Autodesk Fusion 360 part; units mm, degrees
(part 2 of 3)
  spline S11 degree 5 poles (-7.8659, -77.7894) (-7.8562, -77.7792) (-7.8368, -77.7588) (-7.8077, -77.7282) (-7.7692, -77.6872) (-7.7213, -77.6359) (-7.6737, -77.5844) (-7.6264, -77.5328) (-7.5794, -77.481) (-7.5327, -77.4291) (-7.4862, -77.377) (-7.4401, -77.3248) (-7.3942, -77.2724) (-7.3486, -77.2199) (-7.3034, -77.1673) (-7.2584, -77.1145) (-7.2138, -77.0616) (-7.1694, -77.0085) (-7.1254, -76.9553) (-7.0816, -76.9019) (-7.0382, -76.8484) (-6.9951, -76.7947) (-6.9523, -76.7409) (-6.9099, -76.687) (-6.8678, -76.6329) (-6.826, -76.5787) (-6.7845, -76.5243) (-6.7433, -76.4698) (-6.7026, -76.4152) (-6.6621, -76.3604) (-6.622, -76.3054) (-6.5822, -76.2503) (-6.5428, -76.1951) (-6.5038, -76.1397) (-6.4651, -76.0842) (-6.4268, -76.0285) (-6.3888, -75.9727) (-6.3512, -75.9168) (-6.314, -75.8607) (-6.2772, -75.8044) (-6.2407, -75.7481) (-6.2047, -75.6915) (-6.1691, -75.6349) (-6.1338, -75.578) (-6.099, -75.5211) (-6.0646, -75.4639) (-6.0307, -75.4067) (-5.9971, -75.3493) (-5.964, -75.2917) (-5.9313, -75.234) (-5.8991, -75.1761) (-5.8673, -75.1181) (-5.8361, -75.0599) (-5.8054, -75.0016) (-5.7753, -74.9431) (-5.7456, -74.8844) (-5.7163, -74.8256) (-5.6875, -74.7667) (-5.6592, -74.7076) (-5.6315, -74.6483) (-5.6045, -74.5889) (-5.5782, -74.5292) (-5.5528, -74.4693) (-5.5282, -74.4092) (-5.5043, -74.3489) (-5.481, -74.2884) (-5.4581, -74.2278) (-5.4356, -74.1672) (-5.4137, -74.1064) (-5.3929, -74.0453) (-5.3739, -73.9839) (-5.3606, -73.9342) (-5.352, -73.8966) (-5.3468, -73.8714) (-5.3444, -73.8588) knots -1 -1 -1 -1 -1 -1 -0.98571429 -0.97142857 -0.95714286 -0.94285714 -0.92857143 -0.91428571 -0.9 -0.88571429 -0.87142857 -0.85714286 -0.84285714 -0.82857143 -0.81428571 -0.8 -0.78571429 -0.77142857 -0.75714286 -0.74285714 -0.72857143 -0.71428571 -0.7 -0.68571429 -0.67142857 -0.65714286 -0.64285714 -0.62857143 -0.61428571 -0.6 -0.58571429 -0.57142857 -0.55714286 -0.54285714 -0.52857143 -0.51428571 -0.5 -0.48571429 -0.47142857 -0.45714286 -0.44285714 -0.42857143 -0.41428571 -0.4 -0.38571429 -0.37142857 -0.35714286 -0.34285714 -0.32857143 -0.31428571 -0.3 -0.28571429 -0.27142857 -0.25714286 -0.24285714 -0.22857143 -0.21428571 -0.2 -0.18571429 -0.17142857 -0.15714286 -0.14285714 -0.12857143 -0.11428571 -0.1 -0.08571429 -0.07142857 -0.05714286 -0.04285714 -0.02857143 -0.01428571 0 0 0 0 0 0
  line L11 (-5.3444, -73.8588) -> (-5.3408, -73.8396)
  arc A23 (-3.9118, -72.8203) -> (-5.3408, -73.8396) centre (-4.0932, -74.0773) ccw
  arc A24 (-3.9118, -72.8203) -> (-3.2356, -72.9094) centre (0, -45.72) ccw
  arc A25 (-2.1191, -74.2637) -> (-3.2356, -72.9094) centre (-3.3857, -74.1705) ccw
  line L12 (-2.1191, -74.2637) -> (-2.1205, -74.2832)
  spline S12 degree 5 poles (-2.1205, -74.2832) (-2.1215, -74.2961) (-2.1231, -74.3217) (-2.1244, -74.3603) (-2.1245, -74.4117) (-2.122, -74.476) (-2.1177, -74.5403) (-2.1123, -74.6047) (-2.1063, -74.6691) (-2.0998, -74.7335) (-2.093, -74.798) (-2.0855, -74.8624) (-2.0773, -74.9269) (-2.0683, -74.9913) (-2.0583, -75.0557) (-2.0476, -75.1202) (-2.0361, -75.1846) (-2.0241, -75.249) (-2.0115, -75.3134) (-1.9985, -75.3777) (-1.985, -75.4421) (-1.971, -75.5064) (-1.9565, -75.5707) (-1.9414, -75.635) (-1.9257, -75.6992) (-1.9096, -75.7635) (-1.893, -75.8277) (-1.8759, -75.8918) (-1.8583, -75.956) (-1.8403, -76.0201) (-1.8219, -76.0842) (-1.803, -76.1482) (-1.7837, -76.2122) (-1.7639, -76.2762) (-1.7437, -76.3401) (-1.7231, -76.404) (-1.7021, -76.4678) (-1.6807, -76.5317) (-1.6589, -76.5954) (-1.6367, -76.6592) (-1.614, -76.7228) (-1.591, -76.7865) (-1.5677, -76.8501) (-1.5439, -76.9136) (-1.5197, -76.9771) (-1.4952, -77.0406) (-1.4703, -77.104) (-1.4451, -77.1673) (-1.4194, -77.2306) (-1.3935, -77.2939) (-1.3671, -77.3571) (-1.3404, -77.4202) (-1.3134, -77.4833) (-1.286, -77.5464) (-1.2582, -77.6093) (-1.2301, -77.6723) (-1.2017, -77.7351) (-1.1729, -77.7979) (-1.1438, -77.8607) (-1.1144, -77.9234) (-1.0846, -77.986) (-1.0546, -78.0486) (-1.0241, -78.1111) (-0.9934, -78.1735) (-0.9623, -78.2359) (-0.9309, -78.2982) (-0.8992, -78.3605) (-0.8672, -78.4226) (-0.8349, -78.4848) (-0.8022, -78.5468) (-0.7693, -78.6088) (-0.7426, -78.6583) (-0.7225, -78.6954) (-0.7091, -78.7202) (-0.7023, -78.7325) knots 0 0 0 0 0 0 0.01428571 0.02857143 0.04285714 0.05714286 0.07142857 0.08571429 0.1 0.11428571 0.12857143 0.14285714 0.15714286 0.17142857 0.18571429 0.2 0.21428571 0.22857143 0.24285714 0.25714286 0.27142857 0.28571429 0.3 0.31428571 0.32857143 0.34285714 0.35714286 0.37142857 0.38571429 0.4 0.41428571 0.42857143 0.44285714 0.45714286 0.47142857 0.48571429 0.5 0.51428571 0.52857143 0.54285714 0.55714286 0.57142857 0.58571429 0.6 0.61428571 0.62857143 0.64285714 0.65714286 0.67142857 0.68571429 0.7 0.71428571 0.72857143 0.74285714 0.75714286 0.77142857 0.78571429 0.8 0.81428571 0.82857143 0.84285714 0.85714286 0.87142857 0.88571429 0.9 0.91428571 0.92857143 0.94285714 0.95714286 0.97142857 0.98571429 1 1 1 1 1 1
  arc A26 (-0.7023, -78.7325) -> (0.7023, -78.7325) centre (0, -45.72) ccw
  spline S13 degree 5 poles (0.7023, -78.7325) (0.7091, -78.7202) (0.7225, -78.6954) (0.7426, -78.6583) (0.7693, -78.6088) (0.8022, -78.5468) (0.8349, -78.4848) (0.8672, -78.4226) (0.8992, -78.3605) (0.9309, -78.2982) (0.9623, -78.2359) (0.9934, -78.1735) (1.0241, -78.1111) (1.0546, -78.0486) (1.0846, -77.986) (1.1144, -77.9234) (1.1438, -77.8607) (1.1729, -77.7979) (1.2017, -77.7351) (1.2301, -77.6723) (1.2582, -77.6093) (1.286, -77.5464) (1.3134, -77.4833) (1.3404, -77.4202) (1.3671, -77.3571) (1.3935, -77.2939) (1.4194, -77.2306) (1.4451, -77.1673) (1.4703, -77.104) (1.4952, -77.0406) (1.5197, -76.9771) (1.5439, -76.9136) (1.5677, -76.8501) (1.591, -76.7865) (1.614, -76.7228) (1.6367, -76.6592) (1.6589, -76.5954) (1.6807, -76.5317) (1.7021, -76.4678) (1.7231, -76.404) (1.7437, -76.3401) (1.7639, -76.2762) (1.7837, -76.2122) (1.803, -76.1482) (1.8219, -76.0842) (1.8403, -76.0201) (1.8583, -75.956) (1.8759, -75.8918) (1.893, -75.8277) (1.9096, -75.7635) (1.9257, -75.6992) (1.9414, -75.635) (1.9565, -75.5707) (1.971, -75.5064) (1.985, -75.4421) (1.9985, -75.3777) (2.0115, -75.3134) (2.0241, -75.249) (2.0361, -75.1846) (2.0476, -75.1202) (2.0583, -75.0557) (2.0683, -74.9913) (2.0773, -74.9269) (2.0855, -74.8624) (2.093, -74.798) (2.0998, -74.7335) (2.1063, -74.6691) (2.1123, -74.6047) (2.1177, -74.5403) (2.122, -74.476) (2.1245, -74.4117) (2.1244, -74.3603) (2.1231, -74.3217) (2.1215, -74.2961) (2.1205, -74.2832) knots -1 -1 -1 -1 -1 -1 -0.98571429 -0.97142857 -0.95714286 -0.94285714 -0.92857143 -0.91428571 -0.9 -0.88571429 -0.87142857 -0.85714286 -0.84285714 -0.82857143 -0.81428571 -0.8 -0.78571429 -0.77142857 -0.75714286 -0.74285714 -0.72857143 -0.71428571 -0.7 -0.68571429 -0.67142857 -0.65714286 -0.64285714 -0.62857143 -0.61428571 -0.6 -0.58571429 -0.57142857 -0.55714286 -0.54285714 -0.52857143 -0.51428571 -0.5 -0.48571429 -0.47142857 -0.45714286 -0.44285714 -0.42857143 -0.41428571 -0.4 -0.38571429 -0.37142857 -0.35714286 -0.34285714 -0.32857143 -0.31428571 -0.3 -0.28571429 -0.27142857 -0.25714286 -0.24285714 -0.22857143 -0.21428571 -0.2 -0.18571429 -0.17142857 -0.15714286 -0.14285714 -0.12857143 -0.11428571 -0.1 -0.08571429 -0.07142857 -0.05714286 -0.04285714 -0.02857143 -0.01428571 0 0 0 0 0 0
  line L13 (2.1205, -74.2832) -> (2.1191, -74.2637)
  arc A27 (3.2356, -72.9094) -> (2.1191, -74.2637) centre (3.3857, -74.1705) ccw
  arc A28 (3.2356, -72.9094) -> (3.9118, -72.8203) centre (0, -45.72) ccw
  arc A29 (5.3408, -73.8396) -> (3.9118, -72.8203) centre (4.0932, -74.0773) ccw
  line L14 (5.3408, -73.8396) -> (5.3444, -73.8588)
  spline S14 degree 5 poles (5.3444, -73.8588) (5.3468, -73.8714) (5.352, -73.8966) (5.3606, -73.9342) (5.3739, -73.9839) (5.3929, -74.0453) (5.4137, -74.1064) (5.4356, -74.1672) (5.4581, -74.2278) (5.481, -74.2884) (5.5043, -74.3489) (5.5282, -74.4092) (5.5528, -74.4693) (5.5782, -74.5292) (5.6045, -74.5889) (5.6315, -74.6483) (5.6592, -74.7076) (5.6875, -74.7667) (5.7163, -74.8256) (5.7456, -74.8844) (5.7753, -74.9431) (5.8054, -75.0016) (5.8361, -75.0599) (5.8673, -75.1181) (5.8991, -75.1761) (5.9313, -75.234) (5.964, -75.2917) (5.9971, -75.3493) (6.0307, -75.4067) (6.0646, -75.4639) (6.099, -75.5211) (6.1338, -75.578) (6.1691, -75.6349) (6.2047, -75.6915) (6.2407, -75.7481) (6.2772, -75.8044) (6.314, -75.8607) (6.3512, -75.9168) (6.3888, -75.9727) (6.4268, -76.0285) (6.4651, -76.0842) (6.5038, -76.1397) (6.5428, -76.1951) (6.5822, -76.2503) (6.622, -76.3054) (6.6621, -76.3604) (6.7026, -76.4152) (6.7433, -76.4698) (6.7845, -76.5243) (6.826, -76.5787) (6.8678, -76.6329) (6.9099, -76.687) (6.9523, -76.7409) (6.9951, -76.7947) (7.0382, -76.8484) (7.0816, -76.9019) (7.1254, -76.9553) (7.1694, -77.0085) (7.2138, -77.0616) (7.2584, -77.1145) (7.3034, -77.1673) (7.3486, -77.2199) (7.3942, -77.2724) (7.4401, -77.3248) (7.4862, -77.377) (7.5327, -77.4291) (7.5794, -77.481) (7.6264, -77.5328) (7.6737, -77.5844) (7.7213, -77.6359) (7.7692, -77.6872) (7.8077, -77.7282) (7.8368, -77.7588) (7.8562, -77.7792) (7.8659, -77.7894) knots 0 0 0 0 0 0 0.01428571 0.02857143 0.04285714 0.05714286 0.07142857 0.08571429 0.1 0.11428571 0.12857143 0.14285714 0.15714286 0.17142857 0.18571429 0.2 0.21428571 0.22857143 0.24285714 0.25714286 0.27142857 0.28571429 0.3 0.31428571 0.32857143 0.34285714 0.35714286 0.37142857 0.38571429 0.4 0.41428571 0.42857143 0.44285714 0.45714286 0.47142857 0.48571429 0.5 0.51428571 0.52857143 0.54285714 0.55714286 0.57142857 0.58571429 0.6 0.61428571 0.62857143 0.64285714 0.65714286 0.67142857 0.68571429 0.7 0.71428571 0.72857143 0.74285714 0.75714286 0.77142857 0.78571429 0.8 0.81428571 0.82857143 0.84285714 0.85714286 0.87142857 0.88571429 0.9 0.91428571 0.92857143 0.94285714 0.95714286 0.97142857 0.98571429 1 1 1 1 1 1
  arc A30 (7.8659, -77.7894) -> (9.2227, -77.4259) centre (0, -45.72) ccw
  spline S15 degree 5 poles (9.2227, -77.4259) (9.226, -77.4122) (9.2326, -77.3848) (9.2424, -77.3438) (9.2553, -77.289) (9.2711, -77.2206) (9.2866, -77.1522) (9.3017, -77.0839) (9.3166, -77.0155) (9.3311, -76.9472) (9.3453, -76.8789) (9.3591, -76.8106) (9.3727, -76.7423) (9.3859, -76.6741) (9.3987, -76.6058) (9.4113, -76.5376) (9.4235, -76.4695) (9.4354, -76.4013) (9.4469, -76.3332) (9.4581, -76.2651) (9.4689, -76.1971) (9.4794, -76.1291) (9.4896, -76.0611) (9.4994, -75.9932) (9.5088, -75.9253) (9.5179, -75.8574) (9.5266, -75.7896) (9.535, -75.7218) (9.543, -75.6541) (9.5506, -75.5864) (9.5579, -75.5187) (9.5648, -75.4511) (9.5713, -75.3836) (9.5774, -75.3161) (9.5832, -75.2487) (9.5885, -75.1813) (9.5935, -75.114) (9.5981, -75.0468) (9.6023, -74.9796) (9.606, -74.9125) (9.6094, -74.8454) (9.6123, -74.7785) (9.6149, -74.7116) (9.6169, -74.6447) (9.6186, -74.578) (9.6198, -74.5113) (9.6206, -74.4447) (9.621, -74.3782) (9.6209, -74.3118) (9.6204, -74.2455) (9.6193, -74.1793) (9.6178, -74.1132) (9.6157, -74.0472) (9.6131, -73.9813) (9.61, -73.9156) (9.6064, -73.8499) (9.6023, -73.7844) (9.5978, -73.7189) (9.5927, -73.6536) (9.5871, -73.5884) (9.5808, -73.5234) (9.5738, -73.4586) (9.5658, -73.394) (9.5571, -73.3297) (9.5476, -73.2655) (9.5375, -73.2015) (9.5271, -73.1376) (9.5162, -73.0738) (9.5048, -73.0102) (9.4923, -72.9469) (9.478, -72.8842) (9.4647, -72.8345) (9.4534, -72.7977) (9.4452, -72.7733) (9.441, -72.7611) knots -1 -1 -1 -1 -1 -1 -0.98571429 -0.97142857 -0.95714286 -0.94285714 -0.92857143 -0.91428571 -0.9 -0.88571429 -0.87142857 -0.85714286 -0.84285714 -0.82857143 -0.81428571 -0.8 -0.78571429 -0.77142857 -0.75714286 -0.74285714 -0.72857143 -0.71428571 -0.7 -0.68571429 -0.67142857 -0.65714286 -0.64285714 -0.62857143 -0.61428571 -0.6 -0.58571429 -0.57142857 -0.55714286 -0.54285714 -0.52857143 -0.51428571 -0.5 -0.48571429 -0.47142857 -0.45714286 -0.44285714 -0.42857143 -0.41428571 -0.4 -0.38571429 -0.37142857 -0.35714286 -0.34285714 -0.32857143 -0.31428571 -0.3 -0.28571429 -0.27142857 -0.25714286 -0.24285714 -0.22857143 -0.21428571 -0.2 -0.18571429 -0.17142857 -0.15714286 -0.14285714 -0.12857143 -0.11428571 -0.1 -0.08571429 -0.07142857 -0.05714286 -0.04285714 -0.02857143 -0.01428571 0 0 0 0 0 0
  line L15 (9.441, -72.7611) -> (9.4346, -72.7427)
  arc A31 (10.1625, -71.1455) -> (9.4346, -72.7427) centre (10.6338, -72.3248) ccw
  arc A32 (10.1625, -71.1455) -> (10.7926, -70.8845) centre (0, -45.72) ccw
  arc A33 (12.4367, -71.4992) -> (10.7926, -70.8845) centre (11.2931, -72.0517) ccw
  line L16 (12.4367, -71.4992) -> (12.4452, -71.5167)
  spline S16 degree 5 poles (12.4452, -71.5167) (12.4508, -71.5283) (12.4622, -71.5514) (12.4803, -71.5854) (12.506, -71.6299) (12.5403, -71.6844) (12.5762, -71.738) (12.6131, -71.791) (12.6505, -71.8438) (12.6883, -71.8964) (12.7264, -71.9488) (12.7651, -72.0008) (12.8044, -72.0526) (12.8445, -72.1038) (12.8853, -72.1547) (12.9268, -72.2051) (12.969, -72.2551) (13.0116, -72.3049) (13.0546, -72.3544) (13.0981, -72.4036) (13.142, -72.4526) (13.1863, -72.5013) (13.231, -72.5497) (13.2762, -72.5978) (13.3219, -72.6457) (13.368, -72.6932) (13.4145, -72.7405) (13.4614, -72.7875) (13.5087, -72.8343) (13.5563, -72.8808) (13.6043, -72.9271) (13.6527, -72.9731) (13.7014, -73.0189) (13.7505, -73.0644) (13.7999, -73.1097) (13.8497, -73.1547) (13.8998, -73.1995) (13.9503, -73.244) (14.0011, -73.2883) (14.0522, -73.3324) (14.1036, -73.3763) (14.1554, -73.4199) (14.2074, -73.4633) (14.2598, -73.5064) (14.3124, -73.5493) (14.3654, -73.592) (14.4187, -73.6345) (14.4722, -73.6767) (14.5261, -73.7187) (14.5802, -73.7605) (14.6346, -73.8021) (14.6893, -73.8434) (14.7443, -73.8845) (14.7995, -73.9254) (14.855, -73.9661) (14.9108, -74.0065) (14.9669, -74.0468) (15.0232, -74.0868) (15.0797, -74.1266) (15.1366, -74.1661) (15.1937, -74.2055) (15.251, -74.2446) (15.3086, -74.2836) (15.3665, -74.3223) (15.4246, -74.3608) (15.4829, -74.399) (15.5415, -74.4371) (15.6003, -74.4749) (15.6594, -74.5125) (15.7187, -74.55) (15.7782, -74.5872) (15.826, -74.6167) (15.862, -74.6388) (15.886, -74.6535) (15.898, -74.6609) knots 0 0 0 0 0 0 0.01428571 0.02857143 0.04285714 0.05714286 0.07142857 0.08571429 0.1 0.11428571 0.12857143 0.14285714 0.15714286 0.17142857 0.18571429 0.2 0.21428571 0.22857143 0.24285714 0.25714286 0.27142857 0.28571429 0.3 0.31428571 0.32857143 0.34285714 0.35714286 0.37142857 0.38571429 0.4 0.41428571 0.42857143 0.44285714 0.45714286 0.47142857 0.48571429 0.5 0.51428571 0.52857143 0.54285714 0.55714286 0.57142857 0.58571429 0.6 0.61428571 0.62857143 0.64285714 0.65714286 0.67142857 0.68571429 0.7 0.71428571 0.72857143 0.74285714 0.75714286 0.77142857 0.78571429 0.8 0.81428571 0.82857143 0.84285714 0.85714286 0.87142857 0.88571429 0.9 0.91428571 0.92857143 0.94285714 0.95714286 0.97142857 0.98571429 1 1 1 1 1 1
  arc A34 (15.898, -74.6609) -> (17.1145, -73.9585) centre (0, -45.72) ccw
  spline S17 degree 5 poles (17.1145, -73.9585) (17.1142, -73.9444) (17.1134, -73.9163) (17.1123, -73.8741) (17.1106, -73.8179) (17.1081, -73.7477) (17.1054, -73.6777) (17.1023, -73.6077) (17.099, -73.5379) (17.0953, -73.4681) (17.0913, -73.3984) (17.0871, -73.3289) (17.0825, -73.2594) (17.0776, -73.1901) (17.0723, -73.1209) (17.0668, -73.0517) (17.0609, -72.9827) (17.0548, -72.9138) (17.0483, -72.8451) (17.0415, -72.7764) (17.0343, -72.7079) (17.0269, -72.6395) (17.0191, -72.5712) (17.011, -72.503) (17.0025, -72.435) (16.9937, -72.3671) (16.9846, -72.2993) (16.9751, -72.2317) (16.9653, -72.1642) (16.9552, -72.0968) (16.9447, -72.0296) (16.9339, -71.9625) (16.9227, -71.8956) (16.9111, -71.8288) (16.8992, -71.7622) (16.887, -71.6958) (16.8743, -71.6295) (16.8614, -71.5633) (16.848, -71.4974) (16.8343, -71.4315) (16.8202, -71.3659) (16.8057, -71.3005) (16.7908, -71.2352) (16.7755, -71.1701) (16.7599, -71.1052) (16.7438, -71.0405) (16.7273, -70.976) (16.7105, -70.9116) (16.6932, -70.8475) (16.6755, -70.7836) (16.6574, -70.7199) (16.6388, -70.6564) (16.6197, -70.5932) (16.6001, -70.5303) (16.5801, -70.4676) (16.5596, -70.4051) (16.5387, -70.3428) (16.5174, -70.2808) (16.4956, -70.219) (16.4733, -70.1575) (16.4504, -70.0963) (16.4268, -70.0356) (16.4024, -69.9752) (16.3773, -69.9153) (16.3515, -69.8558) (16.3253, -69.7966) (16.2986, -69.7375) (16.2717, -69.6787) (16.2441, -69.6203) (16.2157, -69.5624) (16.1857, -69.5055) (16.16, -69.461) (16.1395, -69.4283) (16.1253, -69.4068) (16.1181, -69.3962) knots -1 -1 -1 -1 -1 -1 -0.98571429 -0.97142857 -0.95714286 -0.94285714 -0.92857143 -0.91428571 -0.9 -0.88571429 -0.87142857 -0.85714286 -0.84285714 -0.82857143 -0.81428571 -0.8 -0.78571429 -0.77142857 -0.75714286 -0.74285714 -0.72857143 -0.71428571 -0.7 -0.68571429 -0.67142857 -0.65714286 -0.64285714 -0.62857143 -0.61428571 -0.6 -0.58571429 -0.57142857 -0.55714286 -0.54285714 -0.52857143 -0.51428571 -0.5 -0.48571429 -0.47142857 -0.45714286 -0.44285714 -0.42857143 -0.41428571 -0.4 -0.38571429 -0.37142857 -0.35714286 -0.34285714 -0.32857143 -0.31428571 -0.3 -0.28571429 -0.27142857 -0.25714286 -0.24285714 -0.22857143 -0.21428571 -0.2 -0.18571429 -0.17142857 -0.15714286 -0.14285714 -0.12857143 -0.11428571 -0.1 -0.08571429 -0.07142857 -0.05714286 -0.04285714 -0.02857143 -0.01428571 0 0 0 0 0 0
  line L17 (16.1181, -69.3962) -> (16.1071, -69.3801)
  arc A35 (16.3968, -67.6489) -> (16.1071, -69.3801) centre (17.1573, -68.666) ccw
  arc A36 (16.3968, -67.6489) -> (16.9379, -67.2337) centre (0, -45.72) ccw
  arc A37 (18.685, -67.4019) -> (16.9379, -67.2337) centre (17.7235, -68.2315) ccw
  line L18 (18.685, -67.4019) -> (18.6978, -67.4167)
  spline S18 degree 5 poles (18.6978, -67.4167) (18.7062, -67.4264) (18.7233, -67.4457) (18.7495, -67.4739) (18.7858, -67.5103) (18.8331, -67.554) (18.8816, -67.5965) (18.931, -67.6382) (18.9808, -67.6795) (19.0309, -67.7205) (19.0813, -67.7612) (19.1321, -67.8015) (19.1835, -67.8413) (19.2355, -67.8804) (19.288, -67.919) (19.3412, -67.9569) (19.3948, -67.9944) (19.4489, -68.0314) (19.5033, -68.068) (19.558, -68.1043) (19.6131, -68.1403) (19.6685, -68.1759) (19.7242, -68.2111) (19.7803, -68.2458) (19.8368, -68.2802) (19.8936, -68.3142) (19.9508, -68.3479) (20.0083, -68.3811) (20.066, -68.4141) (20.1241, -68.4467) (20.1825, -68.4789) (20.2411, -68.5109) (20.3, -68.5425) (20.3592, -68.5738) (20.4187, -68.6047) (20.4784, -68.6353) (20.5384, -68.6656) (20.5987, -68.6956) (20.6592, -68.7252) (20.72, -68.7546) (20.781, -68.7836) (20.8423, -68.8124) (20.9038, -68.8408) (20.9655, -68.8689) (21.0275, -68.8967) (21.0897, -68.9243) (21.1522, -68.9515) (21.2148, -68.9784) (21.2777, -69.0051) (21.3408, -69.0314) (21.4041, -69.0575) (21.4676, -69.0833) (21.5314, -69.1088) (21.5953, -69.134) (21.6595, -69.1589) (21.7238, -69.1835) (21.7884, -69.2079) (21.8531, -69.2319) (21.9181, -69.2557) (21.9832, -69.2792) (22.0486, -69.3025) (22.1141, -69.3254) (22.1798, -69.3481) (22.2457, -69.3705) (22.3118, -69.3927) (22.378, -69.4145) (22.4444, -69.4361) (22.5111, -69.4575) (22.5778, -69.4785) (22.6448, -69.4993) (22.7119, -69.5198) (22.7658, -69.536) (22.8062, -69.5481) (22.8333, -69.556) (22.8468, -69.56) knots 0 0 0 0 0 0 0.01428571 0.02857143 0.04285714 0.05714286 0.07142857 0.08571429 0.1 0.11428571 0.12857143 0.14285714 0.15714286 0.17142857 0.18571429 0.2 0.21428571 0.22857143 0.24285714 0.25714286 0.27142857 0.28571429 0.3 0.31428571 0.32857143 0.34285714 0.35714286 0.37142857 0.38571429 0.4 0.41428571 0.42857143 0.44285714 0.45714286 0.47142857 0.48571429 0.5 0.51428571 0.52857143 0.54285714 0.55714286 0.57142857 0.58571429 0.6 0.61428571 0.62857143 0.64285714 0.65714286 0.67142857 0.68571429 0.7 0.71428571 0.72857143 0.74285714 0.75714286 0.77142857 0.78571429 0.8 0.81428571 0.82857143 0.84285714 0.85714286 0.87142857 0.88571429 0.9 0.91428571 0.92857143 0.94285714 0.95714286 0.97142857 0.98571429 1 1 1 1 1 1
  arc A38 (22.8468, -69.56) -> (23.84, -68.5668) centre (0, -45.72) ccw
  spline S19 degree 5 poles (23.84, -68.5668) (23.836, -68.5533) (23.8281, -68.5262) (23.816, -68.4858) (23.7998, -68.4319) (23.7793, -68.3648) (23.7585, -68.2978) (23.7375, -68.2311) (23.7161, -68.1644) (23.6945, -68.098) (23.6727, -68.0318) (23.6505, -67.9657) (23.6281, -67.8998) (23.6054, -67.8341) (23.5825, -67.7686) (23.5592, -67.7032) (23.5357, -67.6381) (23.5119, -67.5731) (23.4879, -67.5084) (23.4635, -67.4438) (23.4389, -67.3795) (23.414, -67.3153) (23.3888, -67.2514) (23.3633, -67.1876) (23.3375, -67.1241) (23.3114, -67.0608) (23.2851, -66.9977) (23.2584, -66.9348) (23.2315, -66.8722) (23.2043, -66.8097) (23.1767, -66.7475) (23.1489, -66.6855) (23.1208, -66.6238) (23.0924, -66.5623) (23.0636, -66.501) (23.0346, -66.44) (23.0052, -66.3792) (22.9756, -66.3187) (22.9456, -66.2584) (22.9153, -66.1984) (22.8847, -66.1387) (22.8538, -66.0792) (22.8225, -66.02) (22.7909, -65.9611) (22.7589, -65.9025) (22.7267, -65.8441) (22.6941, -65.786) (22.6611, -65.7283) (22.6279, -65.6708) (22.5942, -65.6136) (22.5602, -65.5568) (22.5258, -65.5003) (22.4911, -65.4442) (22.4559, -65.3885) (22.4203, -65.3331) (22.3843, -65.278) (22.348, -65.2233) (22.3114, -65.1689) (22.2744, -65.1148) (22.2369, -65.0612) (22.199, -65.008) (22.1604, -64.9555) (22.1213, -64.9035) (22.0815, -64.8521) (22.0412, -64.8013) (22.0005, -64.7509) (21.9595, -64.7008) (21.9182, -64.651) (21.8765, -64.6016) (21.834, -64.5531) (21.7903, -64.5058) (21.7539, -64.4695) (21.7257, -64.4433) (21.7064, -64.4262) (21.6967, -64.4178) knots -1 -1 -1 -1 -1 -1 -0.98571429 -0.97142857 -0.95714286 -0.94285714 -0.92857143 -0.91428571 -0.9 -0.88571429 -0.87142857 -0.85714286 -0.84285714 -0.82857143 -0.81428571 -0.8 -0.78571429 -0.77142857 -0.75714286 -0.74285714 -0.72857143 -0.71428571 -0.7 -0.68571429 -0.67142857 -0.65714286 -0.64285714 -0.62857143 -0.61428571 -0.6 -0.58571429 -0.57142857 -0.55714286 -0.54285714 -0.52857143 -0.51428571 -0.5 -0.48571429 -0.47142857 -0.45714286 -0.44285714 -0.42857143 -0.41428571 -0.4 -0.38571429 -0.37142857 -0.35714286 -0.34285714 -0.32857143 -0.31428571 -0.3 -0.28571429 -0.27142857 -0.25714286 -0.24285714 -0.22857143 -0.21428571 -0.2 -0.18571429 -0.17142857 -0.15714286 -0.14285714 -0.12857143 -0.11428571 -0.1 -0.08571429 -0.07142857 -0.05714286 -0.04285714 -0.02857143 -0.01428571 0 0 0 0 0 0
  line L19 (21.6967, -64.4178) -> (21.6819, -64.405)
  arc A39 (21.5137, -62.6579) -> (21.6819, -64.405) centre (22.5115, -63.4435) ccw
  arc A40 (21.5137, -62.6579) -> (21.9289, -62.1168) centre (0, -45.72) ccw
  arc A41 (23.6601, -61.8271) -> (21.9289, -62.1168) centre (22.946, -62.8773) ccw
  line L20 (23.6601, -61.8271) -> (23.6762, -61.8381)
  spline S20 degree 5 poles (23.6762, -61.8381) (23.6868, -61.8453) (23.7083, -61.8595) (23.741, -61.88) (23.7855, -61.9057) (23.8424, -61.9357) (23.9003, -61.9641) (23.9587, -61.9917) (24.0175, -62.0186) (24.0766, -62.0453) (24.1358, -62.0715) (24.1953, -62.0973) (24.2552, -62.1224) (24.3156, -62.1468) (24.3763, -62.1704) (24.4375, -62.1933) (24.499, -62.2156) (24.5608, -62.2374) (24.6228, -62.2587) (24.6851, -62.2796) (24.7476, -62.3001) (24.8103, -62.3201) (24.8732, -62.3397) (24.9364, -62.3588) (24.9999, -62.3774) (25.0636, -62.3955) (25.1275, -62.4132) (25.1916, -62.4305) (25.256, -62.4473) (25.3205, -62.4638) (25.3852, -62.4799) (25.4501, -62.4955) (25.5152, -62.5108) (25.5805, -62.5257) (25.6459, -62.5402) (25.7115, -62.5543) (25.7774, -62.568) (25.8433, -62.5814) (25.9095, -62.5943) (25.9758, -62.607) (26.0422, -62.6192) (26.1088, -62.6311) (26.1756, -62.6427) (26.2425, -62.6539) (26.3096, -62.6647) (26.3768, -62.6752) (26.4442, -62.6853) (26.5117, -62.6951) (26.5793, -62.7046) (26.6471, -62.7137) (26.715, -62.7225) (26.783, -62.731) (26.8512, -62.7391) (26.9195, -62.7469) (26.9879, -62.7543) (27.0564, -62.7615) (27.1251, -62.7683) (27.1938, -62.7748) (27.2627, -62.7809) (27.3317, -62.7868) (27.4009, -62.7923) (27.4701, -62.7976) (27.5394, -62.8025) (27.6089, -62.8071) (27.6784, -62.8113) (27.7481, -62.8153) (27.8179, -62.819) (27.8877, -62.8223) (27.9577, -62.8254) (28.0277, -62.8281) (28.0979, -62.8306) (28.1541, -62.8323) (28.1963, -62.8334) (28.2244, -62.8342) (28.2385, -62.8345) knots 0 0 0 0 0 0 0.01428571 0.02857143 0.04285714 0.05714286 0.07142857 0.08571429 0.1 0.11428571 0.12857143 0.14285714 0.15714286 0.17142857 0.18571429 0.2 0.21428571 0.22857143 0.24285714 0.25714286 0.27142857 0.28571429 0.3 0.31428571 0.32857143 0.34285714 0.35714286 0.37142857 0.38571429 0.4 0.41428571 0.42857143 0.44285714 0.45714286 0.47142857 0.48571429 0.5 0.51428571 0.52857143 0.54285714 0.55714286 0.57142857 0.58571429 0.6 0.61428571 0.62857143 0.64285714 0.65714286 0.67142857 0.68571429 0.7 0.71428571 0.72857143 0.74285714 0.75714286 0.77142857 0.78571429 0.8 0.81428571 0.82857143 0.84285714 0.85714286 0.87142857 0.88571429 0.9 0.91428571 0.92857143 0.94285714 0.95714286 0.97142857 0.98571429 1 1 1 1 1 1
  arc A42 (28.2385, -62.8345) -> (28.9409, -61.618) centre (0, -45.72) ccw
  spline S21 degree 5 poles (28.9409, -61.618) (28.9335, -61.606) (28.9188, -61.582) (28.8967, -61.546) (28.8672, -61.4982) (28.83, -61.4387) (28.7925, -61.3794) (28.7549, -61.3203) (28.7171, -61.2615) (28.679, -61.2029) (28.6408, -61.1446) (28.6023, -61.0865) (28.5636, -61.0286) (28.5246, -60.971) (28.4855, -60.9137) (28.4461, -60.8566) (28.4066, -60.7997) (28.3668, -60.7432) (28.3268, -60.6869) (28.2865, -60.6308) (28.2461, -60.575) (28.2054, -60.5195) (28.1645, -60.4643) (28.1234, -60.4093) (28.0821, -60.3546) (28.0405, -60.3002) (27.9987, -60.2461) (27.9567, -60.1922) (27.9145, -60.1387) (27.872, -60.0854) (27.8293, -60.0324) (27.7864, -59.9798) (27.7433, -59.9274) (27.6999, -59.8754) (27.6563, -59.8236) (27.6124, -59.7722) (27.5683, -59.7211) (27.524, -59.6703) (27.4795, -59.6198) (27.4347, -59.5697) (27.3897, -59.5199) (27.3444, -59.4705) (27.2989, -59.4214) (27.2531, -59.3727) (27.2071, -59.3243) (27.1608, -59.2763) (27.1143, -59.2287) (27.0675, -59.1814) (27.0205, -59.1345) (26.9732, -59.088) (26.9257, -59.0419) (26.8778, -58.9962) (26.8297, -58.951) (26.7813, -58.9063) (26.7326, -58.862) (26.6836, -58.8181) (26.6344, -58.7746) (26.5849, -58.7316) (26.5351, -58.689) (26.4851, -58.6468) (26.4347, -58.6053) (26.3838, -58.5645) (26.3326, -58.5244) (26.2808, -58.4851) (26.2288, -58.4464) (26.1764, -58.4083) (26.1238, -58.3705) (26.071, -58.3331) (26.018, -58.2962) (25.9644, -58.2603) (25.9099, -58.226) (25.8654, -58.2003) (25.8314, -58.1822) (25.8083, -58.1708) (25.7967, -58.1652) knots -1 -1 -1 -1 -1 -1 -0.98571429 -0.97142857 -0.95714286 -0.94285714 -0.92857143 -0.91428571 -0.9 -0.88571429 -0.87142857 -0.85714286 -0.84285714 -0.82857143 -0.81428571 -0.8 -0.78571429 -0.77142857 -0.75714286 -0.74285714 -0.72857143 -0.71428571 -0.7 -0.68571429 -0.67142857 -0.65714286 -0.64285714 -0.62857143 -0.61428571 -0.6 -0.58571429 -0.57142857 -0.55714286 -0.54285714 -0.52857143 -0.51428571 -0.5 -0.48571429 -0.47142857 -0.45714286 -0.44285714 -0.42857143 -0.41428571 -0.4 -0.38571429 -0.37142857 -0.35714286 -0.34285714 -0.32857143 -0.31428571 -0.3 -0.28571429 -0.27142857 -0.25714286 -0.24285714 -0.22857143 -0.21428571 -0.2 -0.18571429 -0.17142857 -0.15714286 -0.14285714 -0.12857143 -0.11428571 -0.1 -0.08571429 -0.07142857 -0.05714286 -0.04285714 -0.02857143 -0.01428571 0 0 0 0 0 0
  line L21 (25.7967, -58.1652) -> (25.7792, -58.1567)
  arc A43 (25.1645, -56.5126) -> (25.7792, -58.1567) centre (26.3317, -57.0131) ccw
  arc A44 (25.1645, -56.5126) -> (25.4255, -55.8825) centre (0, -45.72) ccw
  arc A45 (27.0227, -55.1546) -> (25.4255, -55.8825) centre (26.6048, -56.3538) ccw
  line L22 (27.0227, -55.1546) -> (27.0411, -55.161)
  spline S22 degree 5 poles (27.0411, -55.161) (27.0533, -55.1652) (27.0777, -55.1734) (27.1145, -55.1847) (27.1642, -55.198) (27.2269, -55.2123) (27.2902, -55.2248) (27.3538, -55.2362) (27.4176, -55.2471) (27.4815, -55.2575) (27.5455, -55.2676) (27.6097, -55.2771) (27.674, -55.2858) (27.7386, -55.2938) (27.8034, -55.3008) (27.8684, -55.3071) (27.9336, -55.3127) (27.9989, -55.3178) (28.0644, -55.3223) (28.1299, -55.3264) (28.1956, -55.33) (28.2613, -55.3331) (28.3272, -55.3357) (28.3932, -55.3378) (28.4593, -55.3393) (28.5255, -55.3404) (28.5918, -55.3409) (28.6582, -55.341) (28.7247, -55.3406) (28.7913, -55.3398) (28.858, -55.3386) (28.9247, -55.3369) (28.9916, -55.3349) (29.0585, -55.3323) (29.1254, -55.3294) (29.1925, -55.326) (29.2596, -55.3223) (29.3268, -55.3181) (29.394, -55.3135) (29.4613, -55.3085) (29.5287, -55.3032) (29.5961, -55.2974) (29.6636, -55.2913) (29.7311, -55.2848) (29.7987, -55.2779) (29.8664, -55.2706) (29.9341, -55.263) (30.0018, -55.255) (30.0696, -55.2466) (30.1374, -55.2379) (30.2053, -55.2288) (30.2732, -55.2194) (30.3411, -55.2096) (30.4091, -55.1994) (30.4771, -55.1889) (30.5451, -55.1781) (30.6132, -55.1669) (30.6813, -55.1554) (30.7495, -55.1435) (30.8176, -55.1313) (30.8858, -55.1187) (30.9541, -55.1059) (31.0223, -55.0927) (31.0906, -55.0791) (31.1589, -55.0653) (31.2272, -55.0511) (31.2955, -55.0366) (31.3639, -55.0217) (31.4322, -55.0066) (31.5006, -54.9911) (31.569, -54.9753) (31.6238, -54.9624) (31.6648, -54.9526) (31.6922, -54.946) (31.7059, -54.9427) knots 0 0 0 0 0 0 0.01428571 0.02857143 0.04285714 0.05714286 0.07142857 0.08571429 0.1 0.11428571 0.12857143 0.14285714 0.15714286 0.17142857 0.18571429 0.2 0.21428571 0.22857143 0.24285714 0.25714286 0.27142857 0.28571429 0.3 0.31428571 0.32857143 0.34285714 0.35714286 0.37142857 0.38571429 0.4 0.41428571 0.42857143 0.44285714 0.45714286 0.47142857 0.48571429 0.5 0.51428571 0.52857143 0.54285714 0.55714286 0.57142857 0.58571429 0.6 0.61428571 0.62857143 0.64285714 0.65714286 0.67142857 0.68571429 0.7 0.71428571 0.72857143 0.74285714 0.75714286 0.77142857 0.78571429 0.8 0.81428571 0.82857143 0.84285714 0.85714286 0.87142857 0.88571429 0.9 0.91428571 0.92857143 0.94285714 0.95714286 0.97142857 0.98571429 1 1 1 1 1 1
  arc A46 (31.7059, -54.9427) -> (32.0694, -53.5859) centre (0, -45.72) ccw
  spline S23 degree 5 poles (32.0694, -53.5859) (32.0592, -53.5762) (32.0388, -53.5568) (32.0082, -53.5277) (31.9672, -53.4892) (31.9159, -53.4413) (31.8644, -53.3937) (31.8128, -53.3464) (31.761, -53.2994) (31.7091, -53.2527) (31.657, -53.2062) (31.6048, -53.1601) (31.5524, -53.1142) (31.4999, -53.0686) (31.4473, -53.0234) (31.3945, -52.9784) (31.3416, -52.9338) (31.2885, -52.8894) (31.2353, -52.8454) (31.1819, -52.8016) (31.1284, -52.7582) (31.0747, -52.7151) (31.0209, -52.6723) (30.967, -52.6299) (30.9129, -52.5878) (30.8587, -52.546) (30.8043, -52.5045) (30.7498, -52.4633) (30.6952, -52.4226) (30.6404, -52.3821) (30.5854, -52.342) (30.5303, -52.3022) (30.4751, -52.2628) (30.4197, -52.2238) (30.3642, -52.1851) (30.3085, -52.1468) (30.2527, -52.1088) (30.1968, -52.0712) (30.1407, -52.034) (30.0844, -51.9972) (30.0281, -51.9607) (29.9715, -51.9247) (29.9149, -51.8891) (29.858, -51.8538) (29.8011, -51.819) (29.7439, -51.7846) (29.6867, -51.7507) (29.6293, -51.7171) (29.5717, -51.684) (29.514, -51.6513) (29.4561, -51.6191) (29.3981, -51.5873) (29.3399, -51.5561) (29.2816, -51.5254) (29.2231, -51.4953) (29.1644, -51.4656) (29.1056, -51.4363) (29.0467, -51.4075) (28.9876, -51.3792) (28.9283, -51.3515) (28.8689, -51.3245) (28.8092, -51.2982) (28.7493, -51.2728) (28.6892, -51.2482) (28.6289, -51.2243) (28.5684, -51.201) (28.5078, -51.1781) (28.4472, -51.1556) (28.3864, -51.1337) (28.3253, -51.1129) (28.2639, -51.0939) (28.2142, -51.0806) (28.1766, -51.072) (28.1514, -51.0668) (28.1388, -51.0644) knots -1 -1 -1 -1 -1 -1 -0.98571429 -0.97142857 -0.95714286 -0.94285714 -0.92857143 -0.91428571 -0.9 -0.88571429 -0.87142857 -0.85714286 -0.84285714 -0.82857143 -0.81428571 -0.8 -0.78571429 -0.77142857 -0.75714286 -0.74285714 -0.72857143 -0.71428571 -0.7 -0.68571429 -0.67142857 -0.65714286 -0.64285714 -0.62857143 -0.61428571 -0.6 -0.58571429 -0.57142857 -0.55714286 -0.54285714 -0.52857143 -0.51428571 -0.5 -0.48571429 -0.47142857 -0.45714286 -0.44285714 -0.42857143 -0.41428571 -0.4 -0.38571429 -0.37142857 -0.35714286 -0.34285714 -0.32857143 -0.31428571 -0.3 -0.28571429 -0.27142857 -0.25714286 -0.24285714 -0.22857143 -0.21428571 -0.2 -0.18571429 -0.17142857 -0.15714286 -0.14285714 -0.12857143 -0.11428571 -0.1 -0.08571429 -0.07142857 -0.05714286 -0.04285714 -0.02857143 -0.01428571 0 0 0 0 0 0
  line L23 (28.1388, -51.0644) -> (28.1196, -51.0608)
  arc A47 (27.1003, -49.6318) -> (28.1196, -51.0608) centre (28.3573, -49.8132) ccw
  arc A48 (27.1003, -49.6318) -> (27.1894, -48.9556) centre (0, -45.72) ccw
  arc A49 (28.5437, -47.8391) -> (27.1894, -48.9556) centre (28.4505, -49.1057) ccw
  line L24 (28.5437, -47.8391) -> (28.5632, -47.8405)
  spline S24 degree 5 poles (28.5632, -47.8405) (28.5761, -47.8415) (28.6017, -47.8431) (28.6403, -47.8444) (28.6917, -47.8445) (28.756, -47.842) (28.8203, -47.8377) (28.8847, -47.8323) (28.9491, -47.8263) (29.0135, -47.8198) (29.078, -47.813) (29.1424, -47.8055) (29.2069, -47.7973) (29.2713, -47.7883) (29.3357, -47.7783) (29.4002, -47.7676) (29.4646, -47.7561) (29.529, -47.7441) (29.5934, -47.7315) (29.6577, -47.7185) (29.7221, -47.705) (29.7864, -47.691) (29.8507, -47.6765) (29.915, -47.6614) (29.9792, -47.6457) (30.0435, -47.6296) (30.1077, -47.613) (30.1718, -47.5959) (30.236, -47.5783) (30.3001, -47.5603) (30.3642, -47.5419) (30.4282, -47.523) (30.4922, -47.5037) (30.5562, -47.4839) (30.6201, -47.4637) (30.684, -47.4431) (30.7478, -47.4221) (30.8117, -47.4007) (30.8754, -47.3789) (30.9392, -47.3567) (31.0028, -47.334) (31.0665, -47.311) (31.1301, -47.2877) (31.1936, -47.2639) (31.2571, -47.2397) (31.3206, -47.2152) (31.384, -47.1903) (31.4473, -47.1651) (31.5106, -47.1394) (31.5739, -47.1135) (31.6371, -47.0871) (31.7002, -47.0604) (31.7633, -47.0334) (31.8264, -47.006) (31.8893, -46.9782) (31.9523, -46.9501) (32.0151, -46.9217) (32.0779, -46.8929) (32.1407, -46.8638) (32.2034, -46.8344) (32.266, -46.8046) (32.3286, -46.7746) (32.3911, -46.7441) (32.4535, -46.7134) (32.5159, -46.6823) (32.5782, -46.6509) (32.6405, -46.6192) (32.7026, -46.5872) (32.7648, -46.5549) (32.8268, -46.5222) (32.8888, -46.4893) (32.9383, -46.4626) (32.9754, -46.4425) (33.0002, -46.4291) (33.0125, -46.4223) knots 0 0 0 0 0 0 0.01428571 0.02857143 0.04285714 0.05714286 0.07142857 0.08571429 0.1 0.11428571 0.12857143 0.14285714 0.15714286 0.17142857 0.18571429 0.2 0.21428571 0.22857143 0.24285714 0.25714286 0.27142857 0.28571429 0.3 0.31428571 0.32857143 0.34285714 0.35714286 0.37142857 0.38571429 0.4 0.41428571 0.42857143 0.44285714 0.45714286 0.47142857 0.48571429 0.5 0.51428571 0.52857143 0.54285714 0.55714286 0.57142857 0.58571429 0.6 0.61428571 0.62857143 0.64285714 0.65714286 0.67142857 0.68571429 0.7 0.71428571 0.72857143 0.74285714 0.75714286 0.77142857 0.78571429 0.8 0.81428571 0.82857143 0.84285714 0.85714286 0.87142857 0.88571429 0.9 0.91428571 0.92857143 0.94285714 0.95714286 0.97142857 0.98571429 1 1 1 1 1 1
  arc A50 (33.0125, -46.4223) -> (33.0125, -45.0177) centre (0, -45.72) ccw
  spline S25 degree 5 poles (33.0125, -45.0177) (33.0002, -45.0109) (32.9754, -44.9975) (32.9383, -44.9774) (32.8888, -44.9507) (32.8268, -44.9178) (32.7648, -44.8851) (32.7026, -44.8528) (32.6405, -44.8208) (32.5782, -44.7891) (32.5159, -44.7577) (32.4535, -44.7266) (32.3911, -44.6959) (32.3286, -44.6654) (32.266, -44.6354) (32.2034, -44.6056) (32.1407, -44.5762) (32.0779, -44.5471) (32.0151, -44.5183) (31.9523, -44.4899) (31.8893, -44.4618) (31.8264, -44.434) (31.7633, -44.4066) (31.7002, -44.3796) (31.6371, -44.3529) (31.5739, -44.3265) (31.5106, -44.3006) (31.4473, -44.2749) (31.384, -44.2497) (31.3206, -44.2248) (31.2571, -44.2003) (31.1936, -44.1761) (31.1301, -44.1523) (31.0665, -44.129) (31.0028, -44.106) (30.9392, -44.0833) (30.8754, -44.0611) (30.8117, -44.0393) (30.7478, -44.0179) (30.684, -43.9969) (30.6201, -43.9763) (30.5562, -43.9561) (30.4922, -43.9363) (30.4282, -43.917) (30.3642, -43.8981) (30.3001, -43.8797) (30.236, -43.8617) (30.1718, -43.8441) (30.1077, -43.827) (30.0435, -43.8104) (29.9792, -43.7943) (29.915, -43.7786) (29.8507, -43.7635) (29.7864, -43.749) (29.7221, -43.735) (29.6577, -43.7215) (29.5934, -43.7085) (29.529, -43.6959) (29.4646, -43.6839) (29.4002, -43.6724) (29.3357, -43.6617) (29.2713, -43.6517) (29.2069, -43.6427) (29.1424, -43.6345) (29.078, -43.627) (29.0135, -43.6202) (28.9491, -43.6137) (28.8847, -43.6077) (28.8203, -43.6023) (28.756, -43.598) (28.6917, -43.5955) (28.6403, -43.5956) (28.6017, -43.5969) (28.5761, -43.5985) (28.5632, -43.5995) knots -1 -1 -1 -1 -1 -1 -0.98571429 -0.97142857 -0.95714286 -0.94285714 -0.92857143 -0.91428571 -0.9 -0.88571429 -0.87142857 -0.85714286 -0.84285714 -0.82857143 -0.81428571 -0.8 -0.78571429 -0.77142857 -0.75714286 -0.74285714 -0.72857143 -0.71428571 -0.7 -0.68571429 -0.67142857 -0.65714286 -0.64285714 -0.62857143 -0.61428571 -0.6 -0.58571429 -0.57142857 -0.55714286 -0.54285714 -0.52857143 -0.51428571 -0.5 -0.48571429 -0.47142857 -0.45714286 -0.44285714 -0.42857143 -0.41428571 -0.4 -0.38571429 -0.37142857 -0.35714286 -0.34285714 -0.32857143 -0.31428571 -0.3 -0.28571429 -0.27142857 -0.25714286 -0.24285714 -0.22857143 -0.21428571 -0.2 -0.18571429 -0.17142857 -0.15714286 -0.14285714 -0.12857143 -0.11428571 -0.1 -0.08571429 -0.07142857 -0.05714286 -0.04285714 -0.02857143 -0.01428571 0 0 0 0 0 0
  line L25 (28.5632, -43.5995) -> (28.5437, -43.6009)
  arc A51 (27.1894, -42.4844) -> (28.5437, -43.6009) centre (28.4505, -42.3343) ccw
  arc A52 (27.1894, -42.4844) -> (27.1003, -41.8082) centre (0, -45.72) ccw
  arc A53 (28.1196, -40.3792) -> (27.1003, -41.8082) centre (28.3573, -41.6268) ccw
  line L26 (28.1196, -40.3792) -> (28.1388, -40.3756)
  spline S26 degree 5 poles (28.1388, -40.3756) (28.1514, -40.3732) (28.1766, -40.368) (28.2142, -40.3594) (28.2639, -40.3461) (28.3253, -40.3271) (28.3864, -40.3063) (28.4472, -40.2844) (28.5078, -40.2619) (28.5684, -40.239) (28.6289, -40.2157) (28.6892, -40.1918) (28.7493, -40.1672) (28.8092, -40.1418) (28.8689, -40.1155) (28.9283, -40.0885) (28.9876, -40.0608) (29.0467, -40.0325) (29.1056, -40.0037) (29.1644, -39.9744) (29.2231, -39.9447) (29.2816, -39.9146) (29.3399, -39.8839) (29.3981, -39.8527) (29.4561, -39.8209) (29.514, -39.7887) (29.5717, -39.756) (29.6293, -39.7229) (29.6867, -39.6893) (29.7439, -39.6554) (29.8011, -39.621) (29.858, -39.5862) (29.9149, -39.5509) (29.9715, -39.5153) (30.0281, -39.4793) (30.0844, -39.4428) (30.1407, -39.406) (30.1968, -39.3688) (30.2527, -39.3312) (30.3085, -39.2932) (30.3642, -39.2549) (30.4197, -39.2162) (30.4751, -39.1772) (30.5303, -39.1378) (30.5854, -39.098) (30.6404, -39.0579) (30.6952, -39.0174) (30.7498, -38.9767) (30.8043, -38.9355) (30.8587, -38.894) (30.9129, -38.8522) (30.967, -38.8101) (31.0209, -38.7677) (31.0747, -38.7249) (31.1284, -38.6818) (31.1819, -38.6384) (31.2353, -38.5946) (31.2885, -38.5506) (31.3416, -38.5062) (31.3945, -38.4616) (31.4473, -38.4166) (31.4999, -38.3714) (31.5524, -38.3258) (31.6048, -38.2799) (31.657, -38.2338) (31.7091, -38.1873) (31.761, -38.1406) (31.8128, -38.0936) (31.8644, -38.0463) (31.9159, -37.9987) (31.9672, -37.9508) (32.0082, -37.9123) (32.0388, -37.8832) (32.0592, -37.8638) (32.0694, -37.8541) knots 0 0 0 0 0 0 0.01428571 0.02857143 0.04285714 0.05714286 0.07142857 0.08571429 0.1 0.11428571 0.12857143 0.14285714 0.15714286 0.17142857 0.18571429 0.2 0.21428571 0.22857143 0.24285714 0.25714286 0.27142857 0.28571429 0.3 0.31428571 0.32857143 0.34285714 0.35714286 0.37142857 0.38571429 0.4 0.41428571 0.42857143 0.44285714 0.45714286 0.47142857 0.48571429 0.5 0.51428571 0.52857143 0.54285714 0.55714286 0.57142857 0.58571429 0.6 0.61428571 0.62857143 0.64285714 0.65714286 0.67142857 0.68571429 0.7 0.71428571 0.72857143 0.74285714 0.75714286 0.77142857 0.78571429 0.8 0.81428571 0.82857143 0.84285714 0.85714286 0.87142857 0.88571429 0.9 0.91428571 0.92857143 0.94285714 0.95714286 0.97142857 0.98571429 1 1 1 1 1 1
  arc A54 (32.0694, -37.8541) -> (31.7059, -36.4973) centre (0, -45.72) ccw
  spline S27 degree 5 poles (31.7059, -36.4973) (31.6922, -36.494) (31.6648, -36.4874) (31.6238, -36.4776) (31.569, -36.4647) (31.5006, -36.4489) (31.4322, -36.4334) (31.3639, -36.4183) (31.2955, -36.4034) (31.2272, -36.3889) (31.1589, -36.3747) (31.0906, -36.3609) (31.0223, -36.3473) (30.9541, -36.3341) (30.8858, -36.3213) (30.8176, -36.3087) (30.7495, -36.2965) (30.6813, -36.2846) (30.6132, -36.2731) (30.5451, -36.2619) (30.4771, -36.2511) (30.4091, -36.2406) (30.3411, -36.2304) (30.2732, -36.2206) (30.2053, -36.2112) (30.1374, -36.2021) (30.0696, -36.1934) (30.0018, -36.185) (29.9341, -36.177) (29.8664, -36.1694) (29.7987, -36.1621) (29.7311, -36.1552) (29.6636, -36.1487) (29.5961, -36.1426) (29.5287, -36.1368) (29.4613, -36.1315) (29.394, -36.1265) (29.3268, -36.1219) (29.2596, -36.1177) (29.1925, -36.114) (29.1254, -36.1106) (29.0585, -36.1077) (28.9916, -36.1051) (28.9247, -36.1031) (28.858, -36.1014) (28.7913, -36.1002) (28.7247, -36.0994) (28.6582, -36.099) (28.5918, -36.0991) (28.5255, -36.0996) (28.4593, -36.1007) (28.3932, -36.1022) (28.3272, -36.1043) (28.2613, -36.1069) (28.1956, -36.11) (28.1299, -36.1136) (28.0644, -36.1177) (27.9989, -36.1222) (27.9336, -36.1273) (27.8684, -36.1329) (27.8034, -36.1392) (27.7386, -36.1462) (27.674, -36.1542) (27.6097, -36.1629) (27.5455, -36.1724) (27.4815, -36.1825) (27.4176, -36.1929) (27.3538, -36.2038) (27.2902, -36.2152) (27.2269, -36.2277) (27.1642, -36.242) (27.1145, -36.2553) (27.0777, -36.2666) (27.0533, -36.2748) (27.0411, -36.279) knots -1 -1 -1 -1 -1 -1 -0.98571429 -0.97142857 -0.95714286 -0.94285714 -0.92857143 -0.91428571 -0.9 -0.88571429 -0.87142857 -0.85714286 -0.84285714 -0.82857143 -0.81428571 -0.8 -0.78571429 -0.77142857 -0.75714286 -0.74285714 -0.72857143 -0.71428571 -0.7 -0.68571429 -0.67142857 -0.65714286 -0.64285714 -0.62857143 -0.61428571 -0.6 -0.58571429 -0.57142857 -0.55714286 -0.54285714 -0.52857143 -0.51428571 -0.5 -0.48571429 -0.47142857 -0.45714286 -0.44285714 -0.42857143 -0.41428571 -0.4 -0.38571429 -0.37142857 -0.35714286 -0.34285714 -0.32857143 -0.31428571 -0.3 -0.28571429 -0.27142857 -0.25714286 -0.24285714 -0.22857143 -0.21428571 -0.2 -0.18571429 -0.17142857 -0.15714286 -0.14285714 -0.12857143 -0.11428571 -0.1 -0.08571429 -0.07142857 -0.05714286 -0.04285714 -0.02857143 -0.01428571 0 0 0 0 0 0
  line L27 (27.0411, -36.279) -> (27.0227, -36.2854)
  arc A55 (25.4255, -35.5575) -> (27.0227, -36.2854) centre (26.6048, -35.0862) ccw
  arc A56 (25.4255, -35.5575) -> (25.1645, -34.9274) centre (0, -45.72) ccw
  arc A57 (25.7792, -33.2833) -> (25.1645, -34.9274) centre (26.3317, -34.4269) ccw
  line L28 (25.7792, -33.2833) -> (25.7967, -33.2748)
  spline S28 degree 5 poles (25.7967, -33.2748) (25.8083, -33.2692) (25.8314, -33.2578) (25.8654, -33.2397) (25.9099, -33.214) (25.9644, -33.1797) (26.018, -33.1438) (26.071, -33.1069) (26.1238, -33.0695) (26.1764, -33.0317) (26.2288, -32.9936) (26.2808, -32.9549) (26.3326, -32.9156) (26.3838, -32.8755) (26.4347, -32.8347) (26.4851, -32.7932) (26.5351, -32.751) (26.5849, -32.7084) (26.6344, -32.6654) (26.6836, -32.6219) (26.7326, -32.578) (26.7813, -32.5337) (26.8297, -32.489) (26.8778, -32.4438) (26.9257, -32.3981) (26.9732, -32.352) (27.0205, -32.3055) (27.0675, -32.2586) (27.1143, -32.2113) (27.1608, -32.1637) (27.2071, -32.1157) (27.2531, -32.0673) (27.2989, -32.0186) (27.3444, -31.9695) (27.3897, -31.9201) (27.4347, -31.8703) (27.4795, -31.8202) (27.524, -31.7697) (27.5683, -31.7189) (27.6124, -31.6678) (27.6563, -31.6164) (27.6999, -31.5646) (27.7433, -31.5126) (27.7864, -31.4602) (27.8293, -31.4076) (27.872, -31.3546) (27.9145, -31.3013) (27.9567, -31.2478) (27.9987, -31.1939) (28.0405, -31.1398) (28.0821, -31.0854) (28.1234, -31.0307) (28.1645, -30.9757) (28.2054, -30.9205) (28.2461, -30.865) (28.2865, -30.8092) (28.3268, -30.7531) (28.3668, -30.6968) (28.4066, -30.6403) (28.4461, -30.5834) (28.4855, -30.5263) (28.5246, -30.469) (28.5636, -30.4114) (28.6023, -30.3535) (28.6408, -30.2954) (28.679, -30.2371) (28.7171, -30.1785) (28.7549, -30.1197) (28.7925, -30.0606) (28.83, -30.0013) (28.8672, -29.9418) (28.8967, -29.894) (28.9188, -29.858) (28.9335, -29.834) (28.9409, -29.822) knots 0 0 0 0 0 0 0.01428571 0.02857143 0.04285714 0.05714286 0.07142857 0.08571429 0.1 0.11428571 0.12857143 0.14285714 0.15714286 0.17142857 0.18571429 0.2 0.21428571 0.22857143 0.24285714 0.25714286 0.27142857 0.28571429 0.3 0.31428571 0.32857143 0.34285714 0.35714286 0.37142857 0.38571429 0.4 0.41428571 0.42857143 0.44285714 0.45714286 0.47142857 0.48571429 0.5 0.51428571 0.52857143 0.54285714 0.55714286 0.57142857 0.58571429 0.6 0.61428571 0.62857143 0.64285714 0.65714286 0.67142857 0.68571429 0.7 0.71428571 0.72857143 0.74285714 0.75714286 0.77142857 0.78571429 0.8 0.81428571 0.82857143 0.84285714 0.85714286 0.87142857 0.88571429 0.9 0.91428571 0.92857143 0.94285714 0.95714286 0.97142857 0.98571429 1 1 1 1 1 1
  arc A58 (28.9409, -29.822) -> (28.2385, -28.6055) centre (0, -45.72) ccw
  spline S29 degree 5 poles (28.2385, -28.6055) (28.2244, -28.6058) (28.1963, -28.6066) (28.1541, -28.6077) (28.0979, -28.6094) (28.0277, -28.6119) (27.9577, -28.6146) (27.8877, -28.6177) (27.8179, -28.621) (27.7481, -28.6247) (27.6784, -28.6287) (27.6089, -28.6329) (27.5394, -28.6375) (27.4701, -28.6424) (27.4009, -28.6477) (27.3317, -28.6532) (27.2627, -28.6591) (27.1938, -28.6652) (27.1251, -28.6717) (27.0564, -28.6785) (26.9879, -28.6857) (26.9195, -28.6931) (26.8512, -28.7009) (26.783, -28.709) (26.715, -28.7175) (26.6471, -28.7263) (26.5793, -28.7354) (26.5117, -28.7449) (26.4442, -28.7547) (26.3768, -28.7648) (26.3096, -28.7753) (26.2425, -28.7861) (26.1756, -28.7973) (26.1088, -28.8089) (26.0422, -28.8208) (25.9758, -28.833) (25.9095, -28.8457) (25.8433, -28.8586) (25.7774, -28.872) (25.7115, -28.8857) (25.6459, -28.8998) (25.5805, -28.9143) (25.5152, -28.9292) (25.4501, -28.9445) (25.3852, -28.9601) (25.3205, -28.9762) (25.256, -28.9927) (25.1916, -29.0095) (25.1275, -29.0268) (25.0636, -29.0445) (24.9999, -29.0626) (24.9364, -29.0812) (24.8732, -29.1003) (24.8103, -29.1199) (24.7476, -29.1399) (24.6851, -29.1604) (24.6228, -29.1813) (24.5608, -29.2026) (24.499, -29.2244) (24.4375, -29.2467) (24.3763, -29.2696) (24.3156, -29.2932) (24.2552, -29.3176) (24.1953, -29.3427) (24.1358, -29.3685) (24.0766, -29.3947) (24.0175, -29.4214) (23.9587, -29.4483) (23.9003, -29.4759) (23.8424, -29.5043) (23.7855, -29.5343) (23.741, -29.56) (23.7083, -29.5805) (23.6868, -29.5947) (23.6762, -29.6019) knots -1 -1 -1 -1 -1 -1 -0.98571429 -0.97142857 -0.95714286 -0.94285714 -0.92857143 -0.91428571 -0.9 -0.88571429 -0.87142857 -0.85714286 -0.84285714 -0.82857143 -0.81428571 -0.8 -0.78571429 -0.77142857 -0.75714286 -0.74285714 -0.72857143 -0.71428571 -0.7 -0.68571429 -0.67142857 -0.65714286 -0.64285714 -0.62857143 -0.61428571 -0.6 -0.58571429 -0.57142857 -0.55714286 -0.54285714 -0.52857143 -0.51428571 -0.5 -0.48571429 -0.47142857 -0.45714286 -0.44285714 -0.42857143 -0.41428571 -0.4 -0.38571429 -0.37142857 -0.35714286 -0.34285714 -0.32857143 -0.31428571 -0.3 -0.28571429 -0.27142857 -0.25714286 -0.24285714 -0.22857143 -0.21428571 -0.2 -0.18571429 -0.17142857 -0.15714286 -0.14285714 -0.12857143 -0.11428571 -0.1 -0.08571429 -0.07142857 -0.05714286 -0.04285714 -0.02857143 -0.01428571 0 0 0 0 0 0
  line L29 (23.6762, -29.6019) -> (23.6601, -29.6129)
  arc A59 (21.9289, -29.3232) -> (23.6601, -29.6129) centre (22.946, -28.5627) ccw
  arc A60 (21.9289, -29.3232) -> (21.5137, -28.7821) centre (0, -45.72) ccw
  arc A61 (21.6819, -27.035) -> (21.5137, -28.7821) centre (22.5115, -27.9965) ccw
  line L30 (21.6819, -27.035) -> (21.6967, -27.0222)
  spline S30 degree 5 poles (21.6967, -27.0222) (21.7064, -27.0138) (21.7257, -26.9967) (21.7539, -26.9705) (21.7903, -26.9342) (21.834, -26.8869) (21.8765, -26.8384) (21.9182, -26.789) (21.9595, -26.7392) (22.0005, -26.6891) (22.0412, -26.6387) (22.0815, -26.5879) (22.1213, -26.5365) (22.1604, -26.4845) (22.199, -26.432) (22.2369, -26.3788) (22.2744, -26.3252) (22.3114, -26.2711) (22.348, -26.2167) (22.3843, -26.162) (22.4203, -26.1069) (22.4559, -26.0515) (22.4911, -25.9958) (22.5258, -25.9397) (22.5602, -25.8832) (22.5942, -25.8264) (22.6279, -25.7692) (22.6611, -25.7117) (22.6941, -25.654) (22.7267, -25.5959) (22.7589, -25.5375) (22.7909, -25.4789) (22.8225, -25.42) (22.8538, -25.3608) (22.8847, -25.3013) (22.9153, -25.2416) (22.9456, -25.1816) (22.9756, -25.1213) (23.0052, -25.0608) (23.0346, -25) (23.0636, -24.939) (23.0924, -24.8777) (23.1208, -24.8162) (23.1489, -24.7545) (23.1767, -24.6925) (23.2043, -24.6303) (23.2315, -24.5678) (23.2584, -24.5052) (23.2851, -24.4423) (23.3114, -24.3792) (23.3375, -24.3159) (23.3633, -24.2524) (23.3888, -24.1886) (23.414, -24.1247) (23.4389, -24.0605) (23.4635, -23.9962) (23.4879, -23.9316) (23.5119, -23.8669) (23.5357, -23.8019) (23.5592, -23.7368) (23.5825, -23.6714) (23.6054, -23.6059) (23.6281, -23.5402) (23.6505, -23.4743) (23.6727, -23.4082) (23.6945, -23.342) (23.7161, -23.2756) (23.7375, -23.2089) (23.7585, -23.1422) (23.7793, -23.0752) (23.7998, -23.0081) (23.816, -22.9542) (23.8281, -22.9138) (23.836, -22.8867) (23.84, -22.8732) knots 0 0 0 0 0 0 0.01428571 0.02857143 0.04285714 0.05714286 0.07142857 0.08571429 0.1 0.11428571 0.12857143 0.14285714 0.15714286 0.17142857 0.18571429 0.2 0.21428571 0.22857143 0.24285714 0.25714286 0.27142857 0.28571429 0.3 0.31428571 0.32857143 0.34285714 0.35714286 0.37142857 0.38571429 0.4 0.41428571 0.42857143 0.44285714 0.45714286 0.47142857 0.48571429 0.5 0.51428571 0.52857143 0.54285714 0.55714286 0.57142857 0.58571429 0.6 0.61428571 0.62857143 0.64285714 0.65714286 0.67142857 0.68571429 0.7 0.71428571 0.72857143 0.74285714 0.75714286 0.77142857 0.78571429 0.8 0.81428571 0.82857143 0.84285714 0.85714286 0.87142857 0.88571429 0.9 0.91428571 0.92857143 0.94285714 0.95714286 0.97142857 0.98571429 1 1 1 1 1 1
  arc A62 (23.84, -22.8732) -> (22.8468, -21.88) centre (0, -45.72) ccw